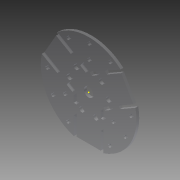
# Autodesk Inventor part: bottom plate
Saved by Autodesk Inventor 2015 (Build 190159000, 159)
## iProperties
Created: 2015-10-18
Part Number: bottom plate
Material: Generic
Document SubType Name: Modeling
Designer: Brian
Density: 1 g/cm^3
Appearance: Polycarbonate - Clear
Mass: 22.7319 g
Surface Area: 175.596 cm^2
Volume: 22.7319 cm^3
Author: Brian
Autodesk Inventor part; units mm, degrees
ref_plane "YZ Plane" through (0, 0, 0) normal (1, 0, 0) x (0, 1, 0)
ref_plane "XZ Plane" through (0, 0, 0) normal (0, 1, 0) x (-1, 0, 0)
ref_plane "XY Plane" through (0, 0, 0) normal (0, 0, 1) x (1, 0, 0)
sketch "Sketch1" plane through (0, 0, 0) normal (0, 1, 0) x (-1, 0, 0)
  circle A0 centre (0, 0) radius 51.5
  dimension "d0" = 103
  constraints: 1 centre point, 1 coincident
  measures "d0" diameter of A0
extrude "Extrusion1" add sketch "Sketch1" along normal blind 3
sketch "Sketch2" plane through (0, 3, 0) normal (0, 1, 0) x (1, 0, 0)
  line L0 (-16, 10.906) -> (16, 10.906) construction
  line L1 (-16, 17.906) -> (16, 17.906) construction
  line L2 (-16, 29.63) -> (16, 29.63) construction
  line L3 (-16, 40) -> (16, 40) construction
  line L4 (16, 10.906) -> (13, 10.906)
  line L5 (13, 10.906) -> (13, 17.906)
  line L6 (13, 17.906) -> (16, 17.906)
  line L7 (16, 17.906) -> (16, 10.906)
  line L8 (16, 29.63) -> (13, 29.63)
  line L9 (13, 29.63) -> (13, 49.8322)
  line L10 (13, 49.8322) -> (16, 49.8322)
  line L11 (16, 49.8322) -> (16, 29.63)
  circle A0 centre (0, 0) radius 51.5 construction
  line L12 (-16, 10.906) -> (-13, 10.906)
  line L13 (-13, 10.906) -> (-13, 17.906)
  line L14 (-13, 17.906) -> (-16, 17.906)
  line L15 (-16, 17.906) -> (-16, 10.906)
  line L16 (-16, 29.63) -> (-13, 29.63)
  line L17 (-13, 29.63) -> (-13, 49.8322)
  line L18 (-13, 49.8322) -> (-16, 49.8322)
  line L19 (-16, 49.8322) -> (-16, 29.63)
  point P0 (0, 10.906)
  dimension "d3" = 10.906
  dimension "d4" = 7
  dimension "d5" = 11.724
  dimension "d6" = 40
  dimension "d7" = 32
  dimension "d8" = 3
  dimension "d9" = 3
  constraints: 40 end point, 10 parallel, 7 vertical alignment, 6 horizontal, 4 perpendicular, 2 collinear, 2 point on circle, 2 point on line, 1 midpoint
  measures "d3" distance from line of point (0, 0) L0
  measures "d4" distance from line of L0 L1.end
  measures "d5" distance between parallel lines of L1 L2
  measures "d6" distance from line of point (0, 0) L3
  measures "d7" distance of L3.start L3.end
  measures "d8" distance of L5.end L6.end
  measures "d9" distance between parallel lines of L15 L13
extrude "Extrusion2" cut sketch "Sketch2" against normal blind 3
sketch "Sketch3" plane through (0, 0, 0) normal (0, -1, 0) x (1, 0, 0)
  circle A0 centre (7.5, -20.006) radius 2.5
  circle A1 centre (-7.5, -20.006) radius 2.5
  line L0 (7.5, -20.006) -> (-7.5, -20.006) construction
  point P0 (0, 0)
  point P1 (0, -20.006)
  dimension "d12" = 5
  dimension "d13" = 15
  dimension "d14" = 20.006
  dimension "d15" = 5
  constraints: 2 centre point, 2 end point, 1 coincident, 1 horizontal, 1 midpoint, 1 vertical alignment
  measures "d12" diameter of A0
  measures "d13" distance of L0.end A0.centre
  measures "d14" vertical distance of point (0, 0) L0.end
  measures "d15" diameter of A1
extrude "Extrusion3" cut sketch "Sketch3" against normal blind 3
sketch "Sketch4" plane through (0, 0, 0) normal (0, -1, 0) x (1, 0, 0)
  circle A0 centre (7.5, -20.006) radius 2.5 construction
  circle A1 centre (-7.5, -20.006) radius 2.5 construction
  line L0 (-13, -29.63) -> (-13, -49.8322) construction
  arc A2 (-13, -49.8322) -> (13, -49.8322) centre (0, 0) ccw construction
  line L1 (13, -49.8322) -> (13, -29.63) construction
  line L2 (13, -29.63) -> (16, -29.63) construction
  line L3 (16, -29.63) -> (16, -48.9515) construction
  arc A3 (16, -48.9515) -> (-16, -48.9515) centre (0, 0) ccw construction
  line L4 (-16, -48.9515) -> (-16, -29.63) construction
  line L5 (-16, -29.63) -> (-13, -29.63) construction
  line L6 (-13, -10.906) -> (-13, -17.906) construction
  line L7 (-13, -17.906) -> (-16, -17.906) construction
  line L8 (-16, -17.906) -> (-16, -10.906) construction
  line L9 (-16, -10.906) -> (-13, -10.906) construction
  line L10 (16, -10.906) -> (16, -17.906) construction
  line L11 (16, -17.906) -> (13, -17.906) construction
  line L12 (13, -17.906) -> (13, -10.906) construction
  line L13 (13, -10.906) -> (16, -10.906) construction
  arc A4 (-13, -49.8322) -> (13, -49.8322) centre (0, 0) ccw projected
  line L14 (13, -48) -> (-13, -48)
  line L15 (-13, -48) -> (-13, -51.5)
  line L16 (-13, -51.5) -> (13, -51.5)
  line L17 (13, -51.5) -> (13, -48)
  line L18 (13, -49.8322) -> (13, -29.63) projected
  line L19 (-13, -29.63) -> (-13, -49.8322) projected
  dimension "d20" = 48
  constraints: 8 end point, 2 collinear, 2 parallel, 1 horizontal, 1 perpendicular, 1 tangent
  measures "d20" distance from line of point (0, 0) L14
extrude "Extrusion4" cut sketch "Sketch4" against normal blind 3
sketch "Sketch5" plane through (0, 0, 0) normal (0, -1, 0) x (1, 0, 0)
  circle A0 centre (0, 0) radius 5
  dimension "d21" = 10
  constraints: 1 centre point, 1 coincident
  measures "d21" diameter of A0
extrude "Extrusion5" cut sketch "Sketch5" against normal blind 3
pattern_circular "Circular Pattern1" count 3 over 360 about axis through (0, 0, 0) along (0, 1, 0) of "Extrusion2", "Extrusion3"
sketch "Sketch6" plane through (0, 0, 0) normal (0, -1, 0) x (1, 0, 0)
  point P0 (0, 0)
pattern_circular "Circular Pattern2" count 3 over 360 about axis through (0, 0, 0) along (0, 1, 0) of "Extrusion4"
sketch "Sketch7" plane through (0, 0, 0) normal (0, -1, 0) x (1, 0, 0)
  circle A0 centre (7.5, -20.006) radius 2.5 construction
  circle A1 centre (-7.5, -20.006) radius 2.5 construction
  line L0 (-13, -10.906) -> (-13, -17.906) construction
  line L1 (-13, -17.906) -> (-16, -17.906) construction
  line L2 (-16, -17.906) -> (-16, -10.906) construction
  line L3 (-16, -10.906) -> (-13, -10.906) construction
  line L4 (16, -10.906) -> (16, -17.906) construction
  line L5 (16, -17.906) -> (13, -17.906) construction
  line L6 (13, -17.906) -> (13, -10.906) construction
  line L7 (13, -10.906) -> (16, -10.906) construction
  circle A2 centre (0, 0) radius 5 construction
  circle A3 centre (-21.0757, 3.5078) radius 2.5 construction
  circle A4 centre (-13.5757, 16.4982) radius 2.5 construction
  line L8 (-2.9449, 16.7113) -> (-9.0071, 20.2113) construction
  line L9 (-9.0071, 20.2113) -> (-7.5071, 22.8094) construction
  line L10 (-7.5071, 22.8094) -> (-1.4449, 19.3094) construction
  line L11 (-1.4449, 19.3094) -> (-2.9449, 16.7113) construction
  line L12 (-17.4449, -8.4034) -> (-23.5071, -4.9034) construction
  line L13 (-23.5071, -4.9034) -> (-22.0071, -2.3053) construction
  line L14 (-22.0071, -2.3053) -> (-15.9449, -5.8053) construction
  line L15 (-15.9449, -5.8053) -> (-17.4449, -8.4034) construction
  circle A5 centre (13.5757, 16.4982) radius 2.5 construction
  circle A6 centre (21.0757, 3.5078) radius 2.5 construction
  line L16 (15.9449, -5.8053) -> (22.0071, -2.3053) construction
  line L17 (22.0071, -2.3053) -> (23.5071, -4.9034) construction
  line L18 (23.5071, -4.9034) -> (17.4449, -8.4034) construction
  line L19 (17.4449, -8.4034) -> (15.9449, -5.8053) construction
  line L20 (1.4449, 19.3094) -> (7.5071, 22.8094) construction
  line L21 (7.5071, 22.8094) -> (9.0071, 20.2113) construction
  line L22 (9.0071, 20.2113) -> (2.9449, 16.7113) construction
  line L23 (2.9449, 16.7113) -> (1.4449, 19.3094) construction
  line L24 (48.0692, 12.7417) -> (35.0692, 35.2583) construction
  line L25 (35.0692, 35.2583) -> (19.1603, 26.0733) construction
  line L26 (19.1603, 26.0733) -> (17.6603, 28.6714) construction
  line L27 (17.6603, 28.6714) -> (34.3932, 38.3322) construction
  arc A7 (34.3932, 38.3322) -> (-34.3932, 38.3322) centre (0, 0) ccw construction
  line L28 (-34.3932, 38.3322) -> (-17.6603, 28.6714) construction
  line L29 (-17.6603, 28.6714) -> (-19.1603, 26.0733) construction
  line L30 (-19.1603, 26.0733) -> (-35.0692, 35.2583) construction
  line L31 (-35.0692, 35.2583) -> (-48.0692, 12.7417) construction
  line L32 (-48.0692, 12.7417) -> (-32.1603, 3.5567) construction
  line L33 (-32.1603, 3.5567) -> (-33.6603, 0.9586) construction
  line L34 (-33.6603, 0.9586) -> (-50.3932, 10.6193) construction
  arc A8 (-50.3932, 10.6193) -> (-16, -48.9515) centre (0, 0) ccw construction
  line L35 (-16, -48.9515) -> (-16, -29.63) construction
  line L36 (-16, -29.63) -> (-13, -29.63) construction
  line L37 (-13, -29.63) -> (-13, -48) construction
  line L38 (-13, -48) -> (13, -48) construction
  line L39 (13, -48) -> (13, -29.63) construction
  line L40 (13, -29.63) -> (16, -29.63) construction
  line L41 (16, -29.63) -> (16, -48.9515) construction
  arc A9 (16, -48.9515) -> (50.3932, 10.6193) centre (0, 0) ccw construction
  line L42 (50.3932, 10.6193) -> (33.6603, 0.9586) construction
  line L43 (33.6603, 0.9586) -> (32.1603, 3.5567) construction
  line L44 (32.1603, 3.5567) -> (48.0692, 12.7417) construction
  line L45 (0, 0) -> (41.5692, 24) construction
  line L46 (35.0692, 35.2583) -> (48.0692, 12.7417) construction
  line L47 (0, 0) -> (-41.5692, 24) construction
  line L48 (0, 0) -> (0, -48) construction
  line L49 (13, -48) -> (-13, -48) construction
  circle A10 centre (0, 0) radius 30 construction
  circle A11 centre (0, 0) radius 45 construction
  line L50 (0, 0) -> (0, 45) construction
  line L51 (0, 0) -> (-22.5, 38.9711) construction
  line L52 (22.5, 38.9711) -> (0, 0) construction
  line L53 (0, 0) -> (-22.5, -38.9711) construction
  line L54 (-45, 0) -> (0, 0) construction
  line L55 (0, 0) -> (45, 0) construction
  line L56 (0, 0) -> (22.5, -38.9711) construction
  line L57 (0, 0) -> (38.9711, -22.5) construction
  line L58 (0, 0) -> (-38.9711, -22.5) construction
  circle A12 centre (0, 45) radius 1.5
  circle A13 centre (-22.5, 38.9711) radius 1.5
  circle A14 centre (22.5, 38.9711) radius 1.5
  circle A15 centre (45, 0) radius 1.5
  circle A16 centre (0, 30) radius 1.5
  circle A17 centre (25.9808, -15) radius 1.5
  circle A18 centre (38.9711, -22.5) radius 1.5
  circle A19 centre (22.5, -38.9711) radius 1.5
  circle A20 centre (-22.5, -38.9711) radius 1.5
  circle A21 centre (-38.9711, -22.5) radius 1.5
  circle A22 centre (-45, 0) radius 1.5
  circle A23 centre (-25.9808, -15) radius 1.5
  dimension "d31" = 90
  dimension "d30" = 60
  dimension "d32" = 30
  dimension "d33" = 30
  dimension "d34" = 30
  dimension "d35" = 30
  dimension "d36" = 30
  dimension "d37" = 30
  dimension "d38" = 120
  dimension "d39" = 120
  dimension "d40" = 3
  dimension "d41" = 3
  dimension "d42" = 3
  dimension "d43" = 3
  dimension "d44" = 3
  dimension "d45" = 3
  dimension "d46" = 3
  dimension "d47" = 3
  dimension "d48" = 3
  dimension "d49" = 3
  dimension "d50" = 3
  dimension "d51" = 3
  constraints: 24 end point, 13 centre point, 11 coincident, 3 midpoint, 3 point on circle, 3 point on line, 1 perpendicular, 1 vertical, 11 other
  measures "d30" diameter of A10
  measures "d32" angle of L48 L53
  measures "d33" angle of L56 L48
  measures "d34" angle of L45 L55
  measures "d35" angle of L52 L45
  measures "d36" angle of L47 L51
  measures "d37" angle of L54 L47
  measures "d38" angle of L57 L58
  measures "d39" angle of L50 L57
  measures "d40" diameter of A12
  measures "d41" diameter of A14
  measures "d42" diameter of A15
  measures "d43" diameter of A16
  measures "d44" diameter of A17
  measures "d45" diameter of A18
  measures "d46" diameter of A19
  measures "d47" diameter of A20
  measures "d48" diameter of A21
  measures "d49" diameter of A22
  measures "d50" diameter of A23
  measures "d51" diameter of A13
extrude "Extrusion6" cut sketch "Sketch7" against normal blind 3
equation "\"d9\" = d8"
equation "\"d15\" = d12"
equation "\"d33\" = d32"
equation "\"d34\" = d32"
equation "\"d35\" = d32"
equation "\"d36\" = d32"
equation "\"d37\" = d32"
equation "\"d41\" = d40"
equation "\"d42\" = d40"
equation "\"d43\" = d40"
equation "\"d44\" = d40"
equation "\"d45\" = d40"
equation "\"d46\" = d40"
equation "\"d47\" = d40"
equation "\"d48\" = d40"
equation "\"d49\" = d40"
equation "\"d50\" = d40"
equation "\"d51\" = d40"
body "Solid1"
